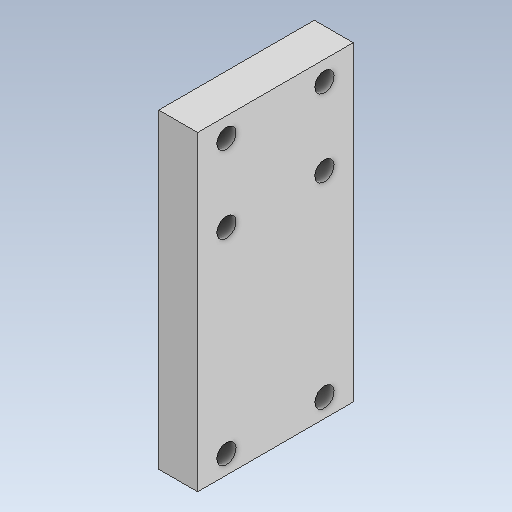
# Autodesk Inventor part: Motor mount
Saved by Autodesk Inventor 2021 (Build 250183000, 183)
## iProperties
Created: 2020-03-13
Part Number: Motor mount
Material: Generic
Document SubType Name: Modeling
Designer: deli
Density: 1 g/cm^3
Appearance: Default
Author: deli
Autodesk Inventor part; units mm, degrees
ref_plane "YZ Plane" through (0, 0, 0) normal (1, 0, 0) x (0, 1, 0)
ref_plane "XZ Plane" through (0, 0, 0) normal (0, 1, 0) x (-1, 0, 0)
ref_plane "XY Plane" through (0, 0, 0) normal (0, 0, 1) x (1, 0, 0)
sketch "Sketch1" plane through (0, 0, 0) normal (1, 0, 0) x (0, 1, 0)
  line L0 (-208.4447, 131.0238) -> (-208.4447, 170.2668) projected
  line L1 (-208.4447, 158.2008) -> (-157.6447, 158.2008)
  line L2 (-157.6447, 158.2008) -> (-157.6447, 132.8008)
  line L3 (-157.6447, 132.8008) -> (-208.4447, 132.8008)
  line L4 (-208.4447, 132.8008) -> (-208.4447, 158.2008)
  circle A0 centre (-205.3947, 153.5008) radius 1.5748
  circle A1 centre (-205.3947, 137.5008) radius 1.5748
  circle A2 centre (-160.8197, 153.5008) radius 1.5748
  circle A3 centre (-160.8197, 137.5008) radius 1.5748
  circle A4 centre (-173.3947, 153.5008) radius 1.5748
  circle A5 centre (-173.3947, 137.5008) radius 1.5748
  point P0 (0, 0)
  dimension "d0" = 50.8
  dimension "d1" = 25.4
  dimension "d2" = 16
  dimension "d4" = 4.7
  dimension "d6" = 3.1496
  dimension "d7" = 0
  dimension "d8" = 3.175
  dimension "d9" = 3.175
  dimension "d10" = 16
  dimension "d13" = 3.1496
  dimension "d14" = 3.1496
  dimension "d15" = 3.1496
  dimension "d16" = 3.1496
  dimension "d17" = 3.1496
  constraints: 8 end point, 6 centre point, 2 parallel, 1 horizontal, 1 perpendicular, 1 point on line
  measures "d0" distance of L2.end L3.end
  measures "d1" distance of L1.end L2.end
  measures "d2" distance of A1.centre A0.centre
  measures "d4" distance from line of L1 A0.centre
  measures "d6" diameter of A2
  measures "d7" vertical distance of A0.centre A2.centre
  measures "d8" distance from line of L2 A2.centre
  measures "d9" distance from line of L2 A3.centre
  measures "d10" distance of A3.centre A2.centre
  measures "d13" diameter of A0
  measures "d14" diameter of A3
  measures "d15" diameter of A1
  measures "d16" diameter of A4
  measures "d17" diameter of A5
extrude "Extrusion1" add sketch "Sketch1" along normal blind 6.35
equation "\"d6\" = d13"
equation "\"d9\" = d8"
equation "\"d10\" = d2"
equation "\"d14\" = d6"
equation "\"d15\" = d13"
equation "\"d16\" = d6"
equation "\"d17\" = d16"
body "Solid1"
